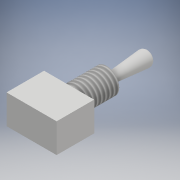
# Autodesk Inventor part: Switch
Saved by Autodesk Inventor 2017 (Build 210142000, 142)
## iProperties
Created: 2017-04-06
Part Number: Switch
Material: Generic
Document SubType Name: Modeling
Designer: AlexS
Density: 1 g/cm^3
Appearance: Default
Author: AlexS
Autodesk Inventor part; units mm, degrees
ref_plane "YZ Plane" through (0, 0, 0) normal (1, 0, 0) x (0, 1, 0)
ref_plane "XZ Plane" through (0, 0, 0) normal (0, 1, 0) x (-1, 0, 0)
ref_plane "XY Plane" through (0, 0, 0) normal (0, 0, 1) x (1, 0, 0)
sketch "Sketch1" plane through (0, 0, 0) normal (0, 1, 0) x (-1, 0, 0)
  line L0 (6, -3.5) -> (-6, -3.5)
  line L1 (-6, -3.5) -> (-6, 3.5)
  line L2 (-6, 3.5) -> (6, 3.5)
  line L3 (6, 3.5) -> (6, -3.5)
  line L4 (6, -3.5) -> (-6, 3.5) construction
  line L5 (-6, -3.5) -> (6, 3.5) construction
  point P0 (0, 0)
  dimension "d0" = 12
  dimension "d1" = 7
  constraints: 12 end point, 2 midpoint, 2 parallel, 1 horizontal, 1 perpendicular
  measures "d0" distance of L1.end L2.end
  measures "d1" distance of L0.end L1.end
extrude "Extrusion1" add sketch "Sketch1" along normal blind 9
sketch "Sketch2" plane through (0, 9, 0) normal (0, 1, 0) x (1, 0, 0)
  circle A0 centre (0, 0) radius 3
  dimension "d4" = 6
  constraints: 1 centre point, 1 coincident
  measures "d4" diameter of A0
extrude "Extrusion2" add sketch "Sketch2" along normal blind 9
sketch "Sketch5" plane through (0, 0, 0) normal (0, 0, 1) x (1, 0, 0)
  line L0 (3, 18) -> (-3, 18) construction
  line L1 (-3, 9) -> (3, 9) construction
  line L2 (0, 18) -> (0, 28)
  line L3 (0, 18) -> (1, 18)
  line L4 (1, 18) -> (1.7768, 26.8789)
  arc A0 (0.8673, 27.9623) -> (0, 28) centre (0, 18) ccw
  arc A1 (0, 28) -> (1.8596, 27.8256) centre (0, 18) ccw construction
  arc A2 (1.7768, 26.8789) -> (0.8673, 27.9623) centre (0.7806, 26.9661) ccw
  point P0 (0, 0)
  dimension "d7" = 10
  dimension "d8" = 1
  dimension "d9" = 85
  dimension "d10" = 1
  constraints: 7 point on circle, 6 end point, 3 centre point, 2 point on line, 2 tangent, 1 coincident, 1 midpoint, 1 vertical
  measures "d7" distance of L2.start L2.end
  measures "d8" distance of L2.start L3.end
  measures "d9" angle of L0 L4
  measures "d10" radius of A2
revolve "Revolution1" add sketch "Sketch5" angle 360 about axis through (0, 18, 0) along (0, 1, 0)
thread "Thread1" size "M6x1" class "6g" standard "ANSI Metric M Profile" full length
body "Solid1"
